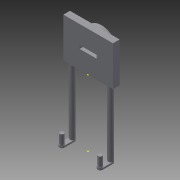
# Autodesk Inventor part: LDR_case
Saved by Autodesk Inventor 2015 SP2 (Build 190223200, 223)
## iProperties
Created: 2016-09-05
Part Number: LDR_case
Material: Generic
Document SubType Name: Modeling
Designer: jm799
Density: 1 g/cm^3
Appearance: Default
Author: jm799
Autodesk Inventor part; units mm, degrees
ref_plane "YZ Plane" through (0, 0, 0) normal (1, 0, 0) x (0, 1, 0)
ref_plane "XZ Plane" through (0, 0, 0) normal (0, 1, 0) x (-1, 0, 0)
ref_plane "XY Plane" through (0, 0, 0) normal (0, 0, 1) x (1, 0, 0)
sketch "Sketch1" plane through (0, 0, 0) normal (0, 1, 0) x (-1, 0, 0)
  line L0 (2.55, 0.5) -> (-2.55, 0.5)
  line L1 (-2.55, 0.5) -> (-2.55, -0.5)
  line L2 (-2.55, -0.5) -> (2.55, -0.5)
  line L3 (2.55, -0.5) -> (2.55, 0.5)
  line L4 (-2.55, 0) -> (2.55, 0) construction
  point P0 (0, 0)
  point P1 (0, -0.5)
  point P2 (0, 0)
  dimension "d0" = 5.1
  dimension "d1" = 1
  constraints: 10 end point, 4 midpoint, 2 parallel, 1 coincident, 1 horizontal, 1 perpendicular
  measures "d0" distance of L2.end L1.end
  measures "d1" distance of L1.end L0.end
sketch "Sketch2" plane through (0, 0, 0) normal (0, 1, 0) x (-1, 0, 0)
  circle A0 centre (0, 0) radius 5
  dimension "d4" = 10
  constraints: 1 centre point, 1 coincident
  measures "d4" diameter of A0
sketch "Sketch3" plane through (0, 0, 0) normal (0, 1, 0) x (-1, 0, 0)
  line L0 (7.5, -6) -> (-7.5, -6)
  line L1 (-7.5, -6) -> (-7.5, 6)
  line L2 (-7.5, 6) -> (7.5, 6)
  line L3 (7.5, 6) -> (7.5, -6)
  line L4 (7.5, 0) -> (-7.5, 0) construction
  line L5 (0, -6) -> (0, 6) construction
  point P0 (0, 0)
  point P1 (0, 0)
  dimension "d2" = 15
  dimension "d3" = 12
  constraints: 12 end point, 5 midpoint, 2 parallel, 1 coincident, 1 horizontal, 1 perpendicular
  measures "d2" distance of L0.start L0.end
  measures "d3" distance of L2.end L0.start
extrude "Extrusion1" add sketch "Sketch3" along normal blind 2
extrude "Extrusion2" cut sketch "Sketch1" along normal blind 2
extrude "Extrusion4" add sketch "Sketch2" along normal blind 4
sketch "Sketch7" plane through (0, 4, 0) normal (0, 1, 0) x (1, 0, 0)
  circle A0 centre (0, 0) radius 4.4878
  constraints: 1 centre point, 1 coincident
extrude "Extrusion5" cut sketch "Sketch7" against normal blind 3
sketch "Sketch8" plane through (0, 1, 0) normal (0, 1, 0) x (1, 0, 0)
  line L0 (-2.55, 0.5) -> (2.55, 0.5)
  line L1 (2.55, 0.5) -> (2.55, -0.5)
  line L2 (2.55, -0.5) -> (-2.55, -0.5)
  line L3 (-2.55, -0.5) -> (-2.55, 0.5)
  line L4 (-2.55, 0) -> (2.55, 0) construction
  line L5 (0, 0.5) -> (0, -0.5) construction
  point P0 (0, 0)
  point P1 (0, 0)
  dimension "d15" = 5.1
  dimension "d16" = 1
  constraints: 12 end point, 5 midpoint, 2 parallel, 1 coincident, 1 horizontal, 1 perpendicular
  measures "d15" distance of L1.end L2.end
  measures "d16" distance of L0.end L1.end
extrude "Extrusion6" cut sketch "Sketch8" against normal blind 3
sketch "Sketch9" plane through (7.5, 0, -6) normal (0, 0, -1) x (-1, 0, 0)
  circle A0 centre (13.2943, 1) radius 0.75
  line L0 (7.5, 0) -> (7.5, 2) construction
  line L1 (2.5, 2) -> (12.5, 2) construction
  circle A1 centre (1.7057, 1) radius 0.75
  dimension "d19" = 1.5
  constraints: 2 centre point, 2 end point, 1 midpoint, 1 symmetric about line, 1 other
  measures "d19" diameter of A0
extrude "Extrusion7" add sketch "Sketch9" along normal blind 20
sketch "Sketch14" plane through (5.7943, 1, -26) normal (0, 0, -1) x (-1, 0, 0)
  circle A0 centre (0, -3.14) radius 0.75
  circle A1 centre (11.5887, -3.14) radius 0.75
  circle A2 centre (11.5887, 0) radius 0.75 projected
  line L0 (10.8387, 0) -> (10.8387, -3.14)
  line L1 (12.3387, 0) -> (12.3387, -3.14)
  circle A3 centre (0, 0) radius 0.75 projected
  line L2 (-0.75, 0) -> (-0.75, -3.14)
  line L3 (0.75, 0) -> (0.75, -3.14)
  point P0 (5.7943, -1)
  dimension "d25" = 1.5
  dimension "d26" = 1.5
  constraints: 8 end point, 8 point on circle, 8 tangent, 2 centre point
  measures "d25" diameter of A0
  measures "d26" diameter of A1
extrude "Extrusion8" add sketch "Sketch14" along normal blind 0.5
sketch "Sketch15" plane through (5.7943, 1, -26) normal (0, 0, 1) x (1, 0, 0)
  point P0 (-5.7943, -1)
sketch "Sketch17" plane through (5.7943, 1, -26) normal (0, 0, 1) x (1, 0, 0)
  line L0 (-13.2943, -1) -> (1.7057, -1) construction
  line L1 (-0.0029, -1) -> (-0.0029, -3.1605) construction
  circle A0 centre (-0.0029, -3.1605) radius 0.6 construction
  line L2 (-5.7943, -1) -> (-5.7943, -3.1605) construction
  circle A1 centre (-0.0029, -3.1605) radius 0.6
  circle A2 centre (-11.5858, -3.1605) radius 0.6 construction
  circle A3 centre (-11.5858, -3.1605) radius 0.6
  circle A4 centre (-0.0029, -3.1605) radius 0.675
  circle A5 centre (-11.5858, -3.1605) radius 0.675
  dimension "d29" = 1.2
  dimension "d32" = 1.35
  dimension "d33" = 1.35
  constraints: 6 centre point, 5 coincident, 4 end point, 2 concentric, 2 vertical, 1 point on line, 1 symmetric about line, 1 other
  measures "d29" diameter of A0
  measures "d32" diameter of A4
  measures "d33" diameter of A5
extrude "Extrusion9" add sketch "Sketch17" along normal blind 3 contours A1 | A3
sketch "Sketch19" plane through (5.7943, 1, -26) normal (0, 0, 1) x (1, 0, 0)
  circle A0 centre (-11.5858, -3.1605) radius 0.6 projected
  circle A1 centre (-11.5858, -3.1605) radius 0.675
  circle A2 centre (-0.0029, -3.1605) radius 0.6 projected
  circle A3 centre (-0.0029, -3.1605) radius 0.675
  point P0 (-5.7943, -1)
  dimension "d34" = 1.35
  dimension "d35" = 1.35
  constraints: 2 centre point, 2 coincident
  measures "d34" diameter of A1
  measures "d35" diameter of A3
extrude "Extrusion10" add sketch "Sketch19" along normal blind 0.25
sketch "Sketch20" plane through (7.5, 0, -6) normal (0, 0, -1) x (-1, 0, 0)
  point P0 (7.5, 0)
body "Solid1"
